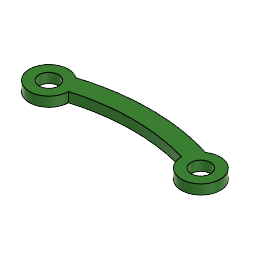
Arm (Autodesk Fusion 360 design; units mm, degrees)
part number: 2026-05-19-18-27-28-641
Autodesk Fusion 360 part; units mm, degrees
sketch "Sketch1" plane through (0, 0, 0) normal (0, 0, 1) x (1, 0, 0)
  circle A0 centre (39, 0) radius 2.5
  circle A1 centre (0, 0) radius 2.5
  arc A2 (34, 0) -> (5, 0) centre (19.5, -48.8953) ccw
  arc A3 (36.0912, 4.0668) -> (2.9088, 4.0668) centre (19.5, -48.8953) ccw
  arc A4 (2.9088, 4.0668) -> (5, 0) centre (0, 0) ccw
  arc A5 (34, 0) -> (36.0912, 4.0668) centre (39, 0) ccw
  dimension "d1" = 39
  dimension "d2" = 5
  dimension "d3" = 10
  dimension "d4" = 5
  dimension "d5" = 10
  dimension "d6" = 51
  dimension "d7" = 4.5
  dimension "d8" = 34
  constraint concentric A0 A5
  constraint coincident A1.centre A4.centre
  constraint concentric A1 A4
  measures "d1" distance of A1.centre A0.centre
  measures "d2" diameter of A0
  measures "d3" diameter of A5
  measures "d4" diameter of A1
  measures "d5" diameter of A4
  measures "d6" radius of A2
  measures "d8" distance of A1.centre A2.start
extrude "Extrude1" add sketch "Sketch1" along normal blind 2.5
